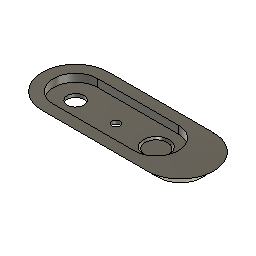
Compact Robot_F2C v1 (Autodesk Fusion 360 design; units mm, degrees)
Autodesk Fusion 360 part; units mm, degrees
sketch "Esboço1" plane through (0, 0, 0) normal (0, 0, 1) x (1, 0, 0)
  line L0 (0, -15) -> (47.41, -15)
  arc A0 (47.41, -15) -> (47.41, 15) centre (47.41, 0) ccw
  line L1 (47.41, 15) -> (0, 15)
  arc A1 (0, 15) -> (0, -15) centre (0, 0) ccw
  line L2 (0, 0) -> (47.41, 0) construction
  line L3 (-15, 0) -> (62.41, 0) construction
  circle A2 centre (0, 0) radius 3.75
  circle A3 centre (18.25, 0) radius 1.875
  dimension "d1" = 15
  dimension "d4" = 77.41
  dimension "d5" = 7.5
  dimension "d6" = 18.25
  dimension "d7" = 3.75
  constraint tangent L0 A0
  constraint tangent A0 L1
  constraint parallel L0 L1
  constraint tangent L1 A1
  constraint tangent L0 A1
  constraint horizontal L2
  constraint coincident A1.centre L2.start
  constraint midpoint A1 L3.start
  constraint midpoint A0 L3.end
  measures "d1" radius of A0
  measures "d4" distance of L3.start L3.end
  measures "d5" diameter of A2
  measures "d6" distance of A1.centre A3.centre
  measures "d7" diameter of A3
extrude "Extrusão1" add sketch "Esboço1" along normal blind 5
sketch "Esboço2" plane through (0, 0, 5) normal (0, 0, 1) x (-1, 0, 0)
  circle A0 centre (-18.25, 0) radius 1.875
  circle A1 centre (0, 0) radius 3.75
  arc A2 (0, -15) -> (0, 15) centre (0, 0) ccw
  line L0 (0, 15) -> (-47.41, 15)
  arc A3 (-47.41, 15) -> (-47.41, -15) centre (-47.41, 0) ccw
  line L1 (-47.41, -15) -> (0, -15)
  line L2 (0, 10) -> (-36.5, 10)
  arc A4 (-36.5, 10) -> (-36.5, -10) centre (-36.5, 0) ccw
  line L3 (-36.5, -10) -> (0, -10)
  arc A5 (0, -10) -> (0, 10) centre (0, 0) ccw
  line L4 (0, 0) -> (-36.5, 0) construction
  dimension "d10" = 36.5
  dimension "d11" = 10
  constraint tangent L2 A4
  constraint tangent A4 L3
  constraint parallel L2 L3
  constraint tangent L3 A5
  constraint tangent L2 A5
  constraint horizontal L4
  constraint coincident A1.centre A2.centre
  measures "d10" distance of A1.centre A4.centre
  measures "d11" radius of A4
extrude "Extrusão2" cut sketch "Esboço2" against normal blind 3.5 contours L2 A4 L3 A5
hole "Furo1" at (36.5, 0, 1.5) direction (0, 0, -1) diameter 10 depth 0.75 tip angle 180
chamfer "Chanfro1" distance 0.75 angle 45 1 edges at (31.8384, 1.8081, 1.5)
chamfer "Chanfro2" distance 5 angle 45 4 edges at (23.705, 15, 0) (-15, 0, 0) (23.705, -15, 0) (62.41, 0, 0)
